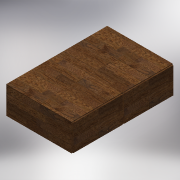
# Autodesk Inventor part: MuebleExtractor
Saved by Autodesk Inventor 2016 (Build 200138000, 138)
## iProperties
Created: 2014-06-18
Part Number: MuebleExtractor
Material: Generic
Document SubType Name: Modeling
Designer: Fernando
Density: 1 g/cm^3
Appearance: Glossy - Black
Sending System: SolidWorks 2014
Last Author: Fernando
Author: Fernando
Autodesk Inventor part; units mm, degrees
ref_plane "YZ Plane" through (0, 0, 0) normal (1, 0, 0) x (0, 1, 0)
ref_plane "XZ Plane" through (0, 0, 0) normal (0, 1, 0) x (-1, 0, 0)
ref_plane "XY Plane" through (0, 0, 0) normal (0, 0, 1) x (1, 0, 0)
ref_plane "Plano de trabajo1" through (-24.9992, 73.6009, 295.6345) normal (0, 1, 0) x (1, 0, 0)
sketch "Boceto1" plane through (-24.9992, 73.6009, 295.6345) normal (0, 1, 0) x (1, 0, 0)
  line L0 (0, -21.25) -> (0, -5.817) projected
  line L1 (0, -21.25) -> (850, -21.25)
  line L2 (850, -21.25) -> (850, 528.929)
  line L3 (850, 528.929) -> (0, 528.929)
  line L4 (0, 528.929) -> (0, -21.25)
  point P0 (24.9992, 295.6345)
  constraints: 8 end point, 2 parallel, 1 horizontal, 1 perpendicular
extrude "Extrusión1" add sketch "Boceto1" along normal blind 302.519
sketch "Boceto2" plane through (-24.9992, 73.6009, 316.8845) normal (0, 0, 1) x (1, 0, 0)
  line L0 (0, 0) -> (850, 0) projected
  line L1 (0, 0) -> (10, 0)
  line L2 (10, 0) -> (10, 10)
  line L3 (0, 302.519) -> (850, 302.519) projected
  line L4 (850, 302.519) -> (840, 302.519)
  line L5 (840, 302.519) -> (840, 292.519)
  line L6 (10, 10) -> (840, 10)
  line L7 (840, 10) -> (840, 292.519)
  line L8 (840, 292.519) -> (10, 292.519)
  line L9 (10, 292.519) -> (10, 10)
  point P0 (24.9992, -73.6009)
  dimension "espesor" = 10
  dimension "d3" = 10
  dimension "d4" = 10
  dimension "d5" = 10
  constraints: 16 end point, 3 perpendicular, 2 parallel, 2 point on line, 1 horizontal
  measures "espesor" distance of L0.start L1.end
  measures "d3" distance of L1.end L2.end
  measures "d4" distance of L3.end L4.end
  measures "d5" distance of L4.end L5.end
extrude "Extrusión2" cut sketch "Boceto2" against normal blind 545
sketch "Boceto3" plane through (-24.9992, 73.6009, 316.8845) normal (0, 0, 1) x (1, 0, 0)
  line L0 (0, 0) -> (5, 0)
  line L1 (850, 0) -> (0, 0) projected
  line L2 (5, 0) -> (5, 5)
  line L3 (0, 302.519) -> (850, 302.519) projected
  line L4 (425, 302.519) -> (420, 302.519)
  line L5 (420, 302.519) -> (420, 297.519)
  line L6 (420, 297.519) -> (5, 297.519)
  line L7 (5, 297.519) -> (5, 5)
  line L8 (5, 5) -> (420, 5)
  line L9 (420, 5) -> (420, 297.519)
  line L10 (425, 302.519) -> (425, 0)
  line L11 (430, 297.519) -> (845, 297.519)
  line L12 (845, 297.519) -> (845, 5)
  line L13 (845, 5) -> (430, 5)
  line L14 (430, 5) -> (430, 297.519)
  point P0 (24.9992, -73.6009)
  dimension "d8" = 5
  dimension "d9" = 5
  dimension "d10" = 5
  dimension "d11" = 5
  constraints: 26 end point, 4 symmetric about line, 3 perpendicular, 2 midpoint, 2 parallel, 2 point on line, 1 horizontal
  measures "d8" distance of L0.start L0.end
  measures "d9" distance of L0.end L2.end
  measures "d10" distance of L4.start L4.end
  measures "d11" distance of L4.end L5.end
extrude "Extrusión3" add sketch "Boceto3" along normal blind 10 contours L7 L6 L9 L8 | L11 L12 L13 L14
sketch "Boceto4" plane through (-24.9992, 73.6009, 326.8845) normal (0, 0, 1) x (1, 0, 0)
  line L0 (5, 5) -> (420, 5) projected
  line L1 (420, 5) -> (420, 297.519) projected
  line L2 (420, 297.519) -> (5, 297.519) projected
  line L3 (5, 297.519) -> (5, 5) projected
  line L4 (845, 297.519) -> (430, 297.519) projected
  line L5 (430, 297.519) -> (430, 5) projected
  line L6 (430, 5) -> (845, 5) projected
  line L7 (845, 5) -> (845, 297.519) projected
  line L8 (10, 10) -> (10, 292.519) projected
  line L9 (10, 35.2519) -> (845, 35.2519) construction
  line L10 (340, 5) -> (340, 297.519) construction
  line L11 (430, 5) -> (845, 5) projected
  line L12 (510, 5) -> (510, 297.519) construction
  circle A0 centre (290, 35.2519) radius 3
  circle A1 centre (390, 35.2519) radius 3
  circle A2 centre (560, 35.2519) radius 3
  circle A3 centre (460, 35.2519) radius 3
  point P0 (24.9992, -73.6009)
  dimension "d15" = 30.2519
  dimension "d16" = 80
  dimension "d17" = 80
  dimension "d18" = 6
  dimension "d19" = 50
  dimension "d20" = 6
  dimension "d21" = 50
  constraints: 8 point on line, 6 end point, 4 centre point, 2 perpendicular, 2 symmetric about line, 1 parallel, 2 other
  measures "d15" distance between parallel lines of L0 L9
  measures "d16" distance between parallel lines of L1 L10
  measures "d17" distance between parallel lines of L12 L5
  measures "d18" diameter of A0
  measures "d19" distance from line of L10 A0.centre
  measures "d20" diameter of A2
  measures "d21" distance from line of L12 A2.centre
extrude "Extrusión4" cut sketch "Boceto4" against normal up to next contours A0 | A1 | A2 | A3
equation "\"d3\" = espesor"
equation "\"d4\" = espesor"
equation "\"d5\" = espesor"
equation "\"d8\" = 0.5 * espesor"
equation "\"d9\" = 0.5 * espesor"
equation "\"d10\" = 0.5 * espesor"
equation "\"d11\" = 0.5 * espesor"
equation "\"d12\" = espesor"
equation "\"d15\" = 0.1 * h_me"
equation "\"h_me\" = 302.519"
